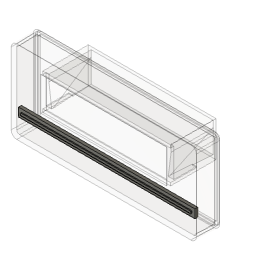
AmigaGotekEnclosure (Autodesk Fusion 360 design; units mm, degrees)
Autodesk Fusion 360 part; units mm, degrees
note: some values were not read from the file. Set by a fixed rule: which face or edge a step refers to.
sketch "Sketch1" plane through (0, 0, 0) normal (0, 1, 0) x (1, 0, 0) in component "face"
  line L0 (77.7875, 34.925) -> (-77.7875, 34.925)
  line L1 (-77.7875, 34.925) -> (-77.7875, -34.925)
  line L2 (-77.7875, -34.925) -> (77.7875, -34.925)
  line L3 (77.7875, -34.925) -> (77.7875, 34.925)
  line L4 (77.7875, 34.925) -> (-77.7875, -34.925) construction
  line L5 (-77.7875, 34.925) -> (77.7875, -34.925) construction
  dimension "d29" = 155.575
  dimension "d30" = 69.85
  constraint horizontal L0
  constraint perpendicular L0 L1
  constraint parallel L0 L2
  constraint parallel L1 L3
  constraint coincident L4 origin
  constraint coincident L5 origin
  measures "d29" distance of L1.end L2.end
  measures "d30" distance of L0.end L1.end
extrude "Extrude1" add sketch "Sketch1" against normal blind 19.05 draft -1 makes body 1 in component "face"
fillet "Fillet1" radius 4.572 4 edges at (-77.6212, -9.525, 34.7587) (77.6212, -9.525, 34.7587) (77.6212, -9.525, -34.7587) (-77.6212, -9.525, -34.7587) on bodies 1 in component "face"
shell "Shell1" thickness 2.3813 removed faces 1 at (-24.4054, 0, -11.6417) on bodies 1 in component "face"
sketch "Sketch2" plane through (0, -19.05, 0) normal (0, -1, 0) x (1, 0, 0) in component "face"
  ellipse E0 centre (-72.8823, -30.0198) end of major axis (-76.1162, -33.2537) minor radius 4.572 (-77.455, -30.0212) -> (-72.8837, -34.5925) ccw
  line L0 (-72.8837, -34.5925) -> (72.8837, -34.5925)
  ellipse E1 centre (72.8823, -30.0198) end of major axis (76.1162, -33.2537) minor radius 4.572 (72.8837, -34.5925) -> (77.455, -30.0212) ccw
  line L1 (77.455, -30.0212) -> (77.455, 30.0212)
  ellipse E2 centre (72.8823, 30.0198) end of major axis (76.1162, 33.2537) minor radius 4.572 (77.455, 30.0212) -> (72.8837, 34.5925) ccw
  line L2 (72.8837, 34.5925) -> (-72.8837, 34.5925)
  ellipse E3 centre (-72.8823, 30.0198) end of major axis (-76.1162, 33.2537) minor radius 4.572 (-72.8837, 34.5925) -> (-77.455, 30.0212) ccw
  line L3 (-77.455, 30.0212) -> (-77.455, -30.0212)
  line L4 (71.4375, -17.5269) -> (-71.4375, -17.5269)
  line L5 (-71.4375, -17.5269) -> (-71.4375, -15.1456)
  line L6 (-71.4375, -15.1456) -> (71.4375, -15.1456)
  line L7 (71.4375, -15.1456) -> (71.4375, -17.5269)
  line L8 (71.4375, -17.5269) -> (-71.4375, -15.1456) construction
  line L9 (-71.4375, -17.5269) -> (71.4375, -15.1456) construction
  line L10 (6.2218, -34.5925) -> (6.2218, -17.5269) construction
  point P0 (0, -16.3362)
  dimension "d36" = 142.875
  dimension "d37" = 2.3813
  dimension "d38" = 17.0656
  constraint horizontal L4
  constraint perpendicular L4 L5
  constraint parallel L4 L6
  constraint parallel L5 L7
  constraint coincident L8 P0
  constraint coincident L9 P0
  constraint coincident L0 L10.start
  constraint coincident L4 L10.end
  constraint perpendicular L4 L10
  measures "d36" distance of L5.end L6.end
  measures "d37" distance of L4.end L5.end
  measures "d38" distance of L10.start L10.end
extrude "Extrude2" cut sketch "Sketch2" against normal up to surface (2.3813 mm away) contours L4 L5 L6 L7 bodies 1 in component "face"
sketch "Sketch3" plane through (0, -16.6688, 0) normal (0, 1, 0) x (-1, 0, 0) in component "face"
  line L0 (-71.4375, -17.5269) -> (-71.4375, -15.1456)
  line L1 (-71.4375, -15.1456) -> (71.4375, -15.1456)
  line L2 (71.4375, -15.1456) -> (71.4375, -17.5269)
  line L3 (71.4375, -17.5269) -> (-71.4375, -17.5269)
  ellipse E0 centre (72.9238, -30.0613) end of major axis (74.4734, -31.6109) minor radius 2.1907 (72.9245, -32.2524) -> (75.1149, -30.062) ccw
  line L4 (75.1149, -30.062) -> (75.1149, 30.062)
  ellipse E1 centre (72.9238, 30.0613) end of major axis (74.4734, 31.6109) minor radius 2.1907 (75.1149, 30.062) -> (72.9245, 32.2524) ccw
  line L5 (72.9245, 32.2524) -> (-72.9245, 32.2524)
  ellipse E2 centre (-72.9238, 30.0613) end of major axis (-74.4734, 31.6109) minor radius 2.1907 (-72.9245, 32.2524) -> (-75.1149, 30.062) ccw
  line L6 (-75.1149, 30.062) -> (-75.1149, -30.062)
  ellipse E3 centre (-72.9238, -30.0613) end of major axis (-74.4734, -31.6109) minor radius 2.1907 (-75.1149, -30.062) -> (-72.9245, -32.2524) ccw
  line L7 (-72.9245, -32.2524) -> (72.9245, -32.2524)
  line L8 (0, -15.1456) -> (0, 32.2524) construction
  line L9 (53.4352, -6.3294) -> (-53.4352, -6.3294)
  line L10 (-53.4352, -6.3294) -> (-53.4352, 23.4362)
  line L11 (-53.4352, 23.4362) -> (53.4353, 23.4362)
  line L12 (53.4353, 23.4362) -> (53.4352, -6.3294)
  line L13 (53.4352, -6.3294) -> (-53.4352, 23.4362) construction
  line L14 (-53.4352, -6.3294) -> (53.4353, 23.4362) construction
  point P0 (0, 8.5534)
  dimension "d42" = 106.8705
  dimension "d43" = 29.7656
  constraint midpoint L1 L8.start
  constraint midpoint L5 L8.end
  constraint horizontal L9
  constraint perpendicular L9 L10
  constraint parallel L9 L11
  constraint parallel L10 L12
  constraint coincident L13 P0
  constraint coincident L14 P0
  constraint midpoint L8 P0
  measures "d42" distance of L10.end L11.end
  measures "d43" distance of L9.end L10.end
extrude "Extrude3" add sketch "Sketch3" along normal blind 38.1 contours L9 L10 L11 L12 bodies 1 in component "face"
shell "Shell2" thickness 2.3813 removed faces 1 at (-17.8118, 21.4312, 13.5144) on bodies 1 in component "face"
ref_plane "WorkPlane4" through (53.4352, 2.3812, 8.5534) normal (1, 0, 0) x (0, 0, -1) in component "face"
sketch "Sketch8" plane through (53.4352, 0, 0) normal (1, 0, 0) x (0, 1, 0) in component "face"
  line L0 (-16.6688, 23.4362) -> (-16.6688, -6.3294)
  line L1 (-16.6688, -6.3294) -> (-16.6688, 23.4362)
  line L2 (-16.6688, -17.5269) -> (-16.6688, -15.1456)
  line L3 (-16.6688, -15.1456) -> (-16.6688, -17.5269)
  line L4 (-16.6688, -32.2524) -> (-16.6688, -30.062)
  line L5 (-16.6688, -30.062) -> (-16.6688, 30.062)
  line L6 (-16.6688, 30.062) -> (-16.6688, 32.2524)
  line L7 (-16.6688, 30.062) -> (-16.6688, 32.2524)
  line L8 (-16.6688, 30.062) -> (-16.6688, -30.062)
  line L9 (-16.6688, -32.2524) -> (-16.6688, -30.062)
  line L10 (-16.6688, -3.9481) -> (21.4312, -3.9481)
  line L11 (21.4312, -3.9481) -> (-16.6688, -3.9481)
  line L12 (-16.6688, 21.055) -> (21.4312, 21.055)
  line L13 (21.4312, 21.055) -> (-16.6688, 21.055)
  line L14 (-16.6688, 21.055) -> (-13.8906, 21.055)
  line L15 (-13.8906, 21.055) -> (-13.8906, -3.9481)
  line L16 (-13.8906, -3.9481) -> (-16.6688, -3.9481)
  line L17 (-16.6688, -3.9481) -> (-16.6688, 21.055)
  dimension "d60" = 2.7781
  constraint horizontal L14
  constraint vertical L15
  constraint horizontal L16
  constraint vertical L17
  constraint coincident L12.start L13.end
  measures "d60" distance of L12.start L14.end
extrude "Extrude6" cut sketch "Sketch8" against normal up to surface (106.8705 mm away) bodies 1 in component "face"
ref_plane "WorkPlane5" through (0, 2.3812, -3.9481) normal (0, 0, 1) x (1, 0, 0) in component "face"
sketch "Sketch9" plane through (0, 0, -3.9481) normal (0, 0, 1) x (1, 0, 0) in component "face"
  line L0 (-51.054, -13.8906) -> (-51.054, 21.4312) construction
  line L1 (-51.054, 21.4312) -> (-51.054, -13.8906) construction
  line L2 (51.054, -13.8906) -> (51.054, 21.4312) construction
  line L3 (51.054, 21.4312) -> (51.054, -13.8906) construction
  line L4 (-51.054, -13.8906) -> (51.054, -13.8906) construction
  line L5 (0, -13.8906) -> (0, 16.5449) construction
  line L6 (-51.054, -13.8906) -> (-48.6728, -13.8906)
  line L7 (-48.6728, -13.8906) -> (-51.054, 21.4312)
  line L8 (-51.054, 21.4312) -> (-51.054, -13.8906)
  line L9 (51.054, -13.8906) -> (48.6727, -13.8906)
  line L10 (48.6727, -13.8906) -> (51.054, 21.4313)
  line L11 (51.054, 21.4313) -> (51.054, -13.8906)
  dimension "d64" = 2.3813
  constraint coincident L0.start L1.end
  constraint coincident L2.start L3.end
  constraint midpoint L4 L5.start
  constraint perpendicular L4 L5
  constraint perpendicular L0 L6
  constraint coincident L0.end L1.start
  constraint symmetric L5 L0.start L2.start
  constraint symmetric L5 L6.end L9.end
  constraint symmetric L5 L0.end L10.end
  measures "d64" distance of L0.start L6.end
extrude "Extrude7" add sketch "Sketch9" along normal up to surface (25.0031 mm away) bodies 1 in component "face"
ref_plane "WorkPlane6" through (-51.054, -13.8906, 8.5534) normal (0, -1, 0) x (0, 0, 1) in component "face"
sketch "Sketch10" plane through (0, -13.8906, 0) normal (0, -1, 0) x (-1, 0, 0) in component "face"
  line L0 (51.054, -21.055) -> (48.6728, -21.055)
  line L1 (48.6728, -21.055) -> (48.6728, 3.9481)
  line L2 (48.6728, 3.9481) -> (51.054, 3.9481)
  line L3 (51.054, 3.9481) -> (51.054, -21.055)
  line L4 (-48.6727, -21.055) -> (-51.054, -21.055)
  line L5 (-51.054, -21.055) -> (-51.054, 3.9481)
  line L6 (-51.054, 3.9481) -> (-48.6727, 3.9481)
  line L7 (-48.6727, 3.9481) -> (-48.6727, -21.055)
  line L8 (51.054, 3.9481) -> (48.6728, 3.9481)
  line L9 (48.6728, 3.9481) -> (53.4352, 3.9481)
  line L10 (53.4352, 3.9481) -> (-53.4352, 3.9481)
  line L11 (-53.4352, 3.9481) -> (-48.6727, 3.9481)
  line L12 (-48.6727, 3.9481) -> (-51.054, 3.9481)
  line L13 (-51.054, 3.9481) -> (51.054, 3.9481)
  line L14 (48.6728, -21.055) -> (51.054, -21.055)
  line L15 (51.054, -21.055) -> (-51.054, -21.055)
  line L16 (-51.054, -21.055) -> (-48.6727, -21.055)
  line L17 (-48.6727, -21.055) -> (-53.4352, -21.055)
  line L18 (-53.4352, -21.055) -> (53.4353, -21.055)
  line L19 (53.4353, -21.055) -> (48.6728, -21.055)
  line L20 (53.4352, 3.9481) -> (53.4353, -21.055)
  line L21 (53.4353, -21.055) -> (53.4353, -23.4362)
  line L22 (53.4353, -23.4362) -> (53.4352, 6.3294)
  line L23 (53.4352, 6.3294) -> (53.4352, 3.9481)
  line L24 (-53.4352, -21.055) -> (-53.4352, 3.9481)
  line L25 (-53.4352, 3.9481) -> (-53.4352, 6.3294)
  line L26 (-53.4352, 6.3294) -> (-53.4352, -23.4362)
  line L27 (-53.4352, -23.4362) -> (-53.4352, -21.055)
  line L28 (48.6728, 3.9481) -> (-48.6727, 3.9481) construction
  line L29 (0, 3.9481) -> (0, -21.055) construction
  line L30 (51.054, 3.9481) -> (51.054, -15.4987) construction
  line L31 (51.054, -15.4987) -> (48.6728, 3.9481)
  line L32 (48.6728, 3.9481) -> (48.6728, -21.055)
  line L33 (48.6728, -21.055) -> (51.054, -21.055)
  line L34 (51.054, -21.055) -> (51.054, -15.4987)
  line L35 (-48.6728, -21.055) -> (-51.054, -21.055)
  line L36 (-48.6727, 3.9481) -> (-48.6728, -21.055)
  line L37 (-51.054, -21.055) -> (-51.054, -15.4987)
  line L38 (-51.054, -15.4987) -> (-48.6727, 3.9481)
  dimension "d68" = 19.4469
  constraint coincident L1.end L2.start
  constraint coincident L6.end L7.start
  constraint midpoint L28 L29.start
  constraint midpoint L18 L29.end
  constraint coincident L2.end L3.start
  constraint perpendicular L8 L30
  constraint coincident L0.end L1.start
  constraint coincident L0.start L3.end
  constraint symmetric L1.end L29 L6.end
  constraint symmetric L29 L30.end L37.end
  constraint symmetric L29 L1.end L6.end
  constraint symmetric L29 L0.end L35.start
  constraint symmetric L29 L0.start L4.end
  measures "d68" distance of L2.end L30.end
extrude "Extrude8" cut sketch "Sketch10" against normal up to surface (35.3219 mm away) contours L0 L1 L3 L14 L15 L18 L19 L31 L32 L33 L34 | L4 L5 L7 L15 L16 L17 L18 L35 L36 L37 L38 bodies 1 in component "face"
sketch "Sketch11" plane through (53.4352, 0, 0) normal (1, 0, 0) x (0, 1, 0) in component "face"
  line L0 (-16.6688, 21.055) -> (-13.8906, 21.055)
  line L1 (-13.8906, 21.055) -> (-13.8906, -3.9481)
  line L2 (-13.8906, -3.9481) -> (-16.6688, -3.9481)
  line L3 (-16.6688, -3.9481) -> (-16.6688, -6.3294)
  line L4 (-16.6688, -6.3294) -> (21.4312, -6.3294)
  line L5 (21.4312, -6.3294) -> (21.4312, 23.4362)
  line L6 (21.4312, 23.4362) -> (-16.6688, 23.4362)
  line L7 (-16.6688, 23.4362) -> (-16.6688, 21.055)
  line L8 (-13.8906, -3.9481) -> (21.4312, -3.9481)
  line L9 (21.4313, -3.9481) -> (-13.8906, -3.9481)
  line L10 (-13.8906, -3.9481) -> (-16.6687, -3.9481)
  line L11 (-16.6688, -3.9481) -> (-13.8906, -3.9481)
  line L12 (-13.8906, 21.055) -> (-13.8906, 15.4987)
  line L13 (-13.8906, 15.4987) -> (-13.8906, -3.9481)
  line L14 (-13.8906, -3.9481) -> (-13.8906, 21.055)
  line L15 (-13.8906, -3.9481) -> (5.1594, -3.9481)
  line L16 (5.1594, -3.9481) -> (5.1594, -3.1544)
  line L17 (5.1594, -3.1544) -> (-13.8906, -3.1544)
  line L18 (-13.8906, -3.1544) -> (-13.8906, -3.9481)
  dimension "d73" = 19.05
  dimension "d74" = 0.7937
  constraint horizontal L15
  constraint vertical L16
  constraint horizontal L17
  constraint vertical L18
  constraint coincident L1.end L2.start
  measures "d73" distance of L1.end L15.end
  measures "d74" distance of L1.end L17.end
extrude "Extrude9" cut sketch "Sketch11" against normal up to surface (106.8705 mm away) contours L1 L8 L9 L13 L14 L15 L16 L17 L18 bodies 1 in component "face"
ref_plane "WorkPlane7" through (0, -16.6688, 0) normal (0, 1, 0) x (1, 0, 0) in component "face"
sketch "Sketch14" plane through (0, -16.6688, 0) normal (0, 1, 0) x (1, 0, 0) in component "face"
  line L0 (51.054, -21.055) -> (51.054, -15.4987)
  line L1 (51.054, -15.4987) -> (51.054, -21.055)
  line L2 (51.054, -21.055) -> (53.4352, -21.055)
  line L3 (53.4352, -21.055) -> (-53.4353, -21.055)
  line L4 (-53.4353, -21.055) -> (-51.054, -21.055)
  line L5 (-51.054, -21.055) -> (51.054, -21.055)
  line L6 (-51.054, -15.4987) -> (-51.054, -21.055)
  line L7 (-51.054, -21.055) -> (-51.054, -15.4987)
  line L8 (49.957, 3.9481) -> (51.054, 3.9481)
  line L9 (51.054, 3.9481) -> (-51.054, 3.9481)
  line L10 (-51.054, 3.9481) -> (-49.957, 3.9481)
  line L11 (-49.957, 3.9481) -> (-53.4352, 3.9481)
  line L12 (-53.4352, 3.9481) -> (53.4352, 3.9481)
  line L13 (53.4352, 3.9481) -> (49.957, 3.9481)
  line L14 (51.054, -21.055) -> (-51.054, -21.055) construction
  line L15 (-51.054, -21.055) -> (-51.054, 3.9481) construction
  line L16 (-51.054, 3.9481) -> (51.054, 3.9481) construction
  line L17 (51.054, 3.9481) -> (51.054, -21.055) construction
  line L18 (-50.2602, -20.2612) -> (-50.2602, 3.1544)
  line L19 (-50.2602, 3.1544) -> (50.2603, 3.1544)
  line L20 (50.2603, 3.1544) -> (50.2603, -20.2612)
  line L21 (50.2603, -20.2612) -> (-50.2602, -20.2612)
  dimension "d81" = 0.7937
  constraint horizontal L14
  constraint vertical L15
  constraint horizontal L16
  constraint vertical L17
  constraint coincident L9.end L10.start
  constraint coincident L0.start L1.end
extrude "Extrude10" cut sketch "Sketch14" against normal up to surface (2.3812 mm away) bodies 1 in component "face"
ref_plane "WorkPlane8" through (0, 0, 0) normal (1, 0, 0) x (0, 1, 0) in component "face"
sketch "Sketch15" plane through (0, 0, 0) normal (1, 0, 0) x (0, 1, 0) in component "face"
  line L0 (-19.05, -3.1544) -> (-16.6688, -3.1544)
  line L1 (-16.6688, -3.1544) -> (-19.05, -3.1544)
  line L2 (-16.6688, 20.2612) -> (-16.6688, -3.1544)
  line L3 (-16.6688, -3.1544) -> (-16.6688, 20.2612)
  line L4 (-16.6688, -3.9481) -> (-16.6688, -6.3294)
  line L5 (-16.6688, -6.3294) -> (-16.6688, -3.9481)
  line L6 (-16.6688, -32.2524) -> (-16.6688, -30.062)
  line L7 (-16.6688, -30.062) -> (-16.6688, 30.062)
  line L8 (-16.6688, 30.062) -> (-16.6688, 32.2524)
  line L9 (-16.6688, 30.062) -> (-16.6688, 32.2524)
  line L10 (-16.6688, 30.062) -> (-16.6688, -30.062)
  line L11 (-16.6688, -32.2524) -> (-16.6688, -30.062)
  line L12 (-16.6688, -17.5269) -> (-16.6688, -15.1456)
  line L13 (-16.6688, -15.1456) -> (-16.6688, -17.5269)
  line L14 (-16.6688, 21.055) -> (-16.6688, 23.4362)
  line L15 (-16.6688, 23.4362) -> (-16.6688, 21.055)
  line L16 (-16.6688, -3.1544) -> (-19.05, -3.1544)
  line L17 (-19.05, -3.1544) -> (-19.05, -5.5356)
  line L18 (-19.05, -5.5356) -> (-16.6688, -3.1544)
  constraint coincident L0.end L1.start
  constraint coincident L0.start L1.end
  constraint perpendicular L1 L17
  constraint equal L16 L17
sweep "Sweep1" cut profiles "Sketch15" along 4 edges at (0, -16.6688, 20.2612) (-50.2602, -16.6688, 8.5534) (0, -16.6688, -3.1544) (50.2603, -16.6688, 8.5534) section 1 on bodies 1 bodies 1 in component "face"
sketch "Sketch16" plane through (0, 0, 0) normal (0, 1, 0) x (-1, 0, 0) in component "face"
  ellipse E0 centre (73.2148, -30.3523) end of major axis (74.7644, -31.9019) minor radius 2.1907 (73.2155, -32.5434) -> (75.4059, -30.353) ccw
  line L0 (73.2155, -32.5434) -> (-73.2155, -32.5434)
  ellipse E1 centre (-73.2148, -30.3523) end of major axis (-74.7644, -31.9019) minor radius 2.1907 (-75.4059, -30.353) -> (-73.2155, -32.5434) ccw
  line L1 (-75.4059, -30.353) -> (-75.4059, 30.353)
  ellipse E2 centre (-73.2148, 30.3523) end of major axis (-74.7644, 31.9019) minor radius 2.1907 (-73.2155, 32.5434) -> (-75.4059, 30.353) ccw
  line L2 (-73.2155, 32.5434) -> (73.2155, 32.5434)
  ellipse E3 centre (73.2148, 30.3523) end of major axis (74.7644, 31.9019) minor radius 2.1907 (75.4059, 30.353) -> (73.2155, 32.5434) ccw
  line L3 (75.4059, 30.353) -> (75.4059, -30.353)
  ellipse E4 centre (73.2148, -30.3523) end of major axis (76.4487, -33.5862) minor radius 4.572 (73.2162, -34.925) -> (77.7875, -30.3537) ccw
  line L4 (77.7875, -30.3537) -> (77.7875, 30.3537)
  ellipse E5 centre (73.2148, 30.3523) end of major axis (76.4487, 33.5862) minor radius 4.572 (77.7875, 30.3537) -> (73.2162, 34.925) ccw
  line L5 (73.2162, 34.925) -> (-73.2162, 34.925)
  ellipse E6 centre (-73.2148, 30.3523) end of major axis (-76.4487, 33.5862) minor radius 4.572 (-73.2162, 34.925) -> (-77.7875, 30.3537) ccw
  line L6 (-77.7875, 30.3537) -> (-77.7875, -30.3537)
  ellipse E7 centre (-73.2148, -30.3523) end of major axis (-76.4487, -33.5862) minor radius 4.572 (-77.7875, -30.3537) -> (-73.2162, -34.925) ccw
  line L7 (-73.2162, -34.925) -> (73.2162, -34.925)
  line L8 (-77.7875, 30.3537) -> (-77.7875, -30.3537)
  ellipse E8 centre (-73.2148, 30.3523) end of major axis (-76.4487, 33.5862) minor radius 4.572 (-73.2162, 34.925) -> (-77.7875, 30.3537) ccw
  line L9 (73.2162, 34.925) -> (-73.2162, 34.925)
  ellipse E9 centre (-73.2148, -30.3523) end of major axis (-76.4487, -33.5862) minor radius 4.572 (-77.7875, -30.3537) -> (-73.2162, -34.925) ccw
  line L10 (-73.2162, -34.925) -> (73.2162, -34.925)
  ellipse E10 centre (73.2148, -30.3523) end of major axis (76.4487, -33.5862) minor radius 4.572 (73.2162, -34.925) -> (77.7875, -30.3537) ccw
  line L11 (77.7875, -30.3537) -> (77.7875, 30.3537)
  ellipse E11 centre (73.2148, 30.3523) end of major axis (76.4487, 33.5862) minor radius 4.572 (77.7875, 30.3537) -> (73.2162, 34.925) ccw
  line L12 (-73.2162, -33.3375) -> (73.2162, -33.3375)
  spline S0 degree 3 poles (73.2162, -33.3375) (74.2378, -33.3375) (75.241, -32.7718) (75.7695, -31.8978) (76.0494, -31.435) (76.2, -30.8948) (76.2, -30.3537) knots -0.785246 -0.785246 -0.785246 -0.785246 0.241471 0.241471 0.241471 0.785246 0.785246 0.785246 0.785246
  line L13 (76.2, -30.3537) -> (76.2, 30.3537)
  spline S1 degree 3 poles (76.2, 30.3537) (76.2, 31.3753) (75.6343, 32.3785) (74.7603, 32.907) (74.2975, 33.1869) (73.7573, 33.3375) (73.2162, 33.3375) knots -0.785246 -0.785246 -0.785246 -0.785246 0.241471 0.241471 0.241471 0.785246 0.785246 0.785246 0.785246
  line L14 (73.2162, 33.3375) -> (-73.2162, 33.3375)
  spline S2 degree 3 poles (-73.2162, 33.3375) (-74.2378, 33.3375) (-75.241, 32.7718) (-75.7695, 31.8978) (-76.0494, 31.435) (-76.2, 30.8948) (-76.2, 30.3537) knots -0.785246 -0.785246 -0.785246 -0.785246 0.241471 0.241471 0.241471 0.785246 0.785246 0.785246 0.785246
  line L15 (-76.2, 30.3537) -> (-76.2, -30.3537)
  spline S3 degree 3 poles (-76.2, -30.3537) (-76.2, -31.3753) (-75.6343, -32.3785) (-74.7603, -32.907) (-74.2975, -33.1869) (-73.7573, -33.3375) (-73.2162, -33.3375) knots -0.785246 -0.785246 -0.785246 -0.785246 0.241471 0.241471 0.241471 0.785246 0.785246 0.785246 0.785246
  line L16 (-73.2162, -30.9562) -> (73.2162, -30.9562)
  spline S4 degree 3 poles (73.2162, -30.9562) (73.5324, -30.9562) (73.8188, -30.6699) (73.8188, -30.3537) knots -0.785246 -0.785246 -0.785246 -0.785246 0.785246 0.785246 0.785246 0.785246
  line L17 (73.8188, -30.3537) -> (73.8188, 30.3537)
  spline S5 degree 3 poles (73.8188, 30.3537) (73.8188, 30.6699) (73.5324, 30.9562) (73.2162, 30.9562) knots -0.785246 -0.785246 -0.785246 -0.785246 0.785246 0.785246 0.785246 0.785246
  line L18 (73.2162, 30.9562) -> (-73.2162, 30.9562)
  spline S6 degree 3 poles (-73.2162, 30.9562) (-73.5324, 30.9562) (-73.8188, 30.6699) (-73.8188, 30.3537) knots -0.785246 -0.785246 -0.785246 -0.785246 0.785246 0.785246 0.785246 0.785246
  line L19 (-73.8188, 30.3537) -> (-73.8188, -30.3537)
  spline S7 degree 3 poles (-73.8188, -30.3537) (-73.8188, -30.6699) (-73.5324, -30.9562) (-73.2162, -30.9562) knots -0.785246 -0.785246 -0.785246 -0.785246 0.785246 0.785246 0.785246 0.785246
extrude "Extrude12" add sketch "Sketch16" along normal blind 1.5875 contours E0 L0 E1 L1 E2 L2 E3 L3 | L12 S0 L13 S1 L14 S2 L15 S3 bodies 1 in component "face"
sketch "Sketch17" plane through (53.4352, 0, 0) normal (1, 0, 0) x (0, 1, 0) in component "face"
  line L0 (0, -30.9563) -> (0, -30.3537)
  line L1 (0, -30.3537) -> (0, -30.9563)
  line L2 (0, -30.3537) -> (0, 30.3537)
  line L3 (0, 30.9563) -> (0, 30.3537)
  line L4 (0, 30.3537) -> (0, 30.9563)
  line L5 (0, 30.3537) -> (0, -30.3537)
  line L6 (0, -30.353) -> (0, -32.5434)
  line L7 (0, -30.353) -> (0, -32.5434)
  line L8 (0, -30.353) -> (0, 30.353)
  line L9 (0, 32.5434) -> (0, 30.353)
  line L10 (0, 32.5434) -> (0, 30.353)
  line L11 (0, 30.353) -> (0, -30.353)
  line L12 (0, -32.5434) -> (-16.6688, -32.2524)
  line L13 (-16.6688, -32.2524) -> (0, -32.5434)
  line L14 (0, -30.9563) -> (0, -32.5434)
  line L15 (0, -32.5434) -> (-1.5869, -32.5157)
  line L16 (0, -30.9563) -> (-1.5869, -32.5157)
  constraint coincident L0.start L1.end
  constraint coincident L6.end L7.end
  constraint coincident L13 L15.end
  constraint parallel L13 L15
  constraint equal L14 L15
sweep "Sweep2" add profiles "Sketch17" along 8 edges at (75.4059, 0, 0) (74.7644, 0, 31.9019) (0, 0, 32.5434) (-74.7644, 0, 31.9019) (-75.4059, 0, 0) (-74.7644, 0, -31.9019) (0, 0, -32.5434) (74.7644, 0, -31.9019) section 1 on bodies 1 bodies 1 in component "face"
sketch "Sketch1 (2)" plane through (0, -16.6688, 0) normal (0, 1, 0) x (-1, 0, 0) in component "accent_line"
  line L0 (-50.2603, 20.2612) -> (50.2602, 20.2612)
  line L1 (50.2602, 20.2612) -> (50.2602, -3.1544)
  line L2 (50.2602, -3.1544) -> (-50.2603, -3.1544)
  line L3 (-50.2603, -3.1544) -> (-50.2603, 20.2612)
  line L4 (-53.4352, -3.9481) -> (53.4352, -3.9481)
  line L5 (53.4352, -3.9481) -> (53.4352, -6.3294)
  line L6 (53.4352, -6.3294) -> (-53.4352, -6.3294)
  line L7 (-53.4352, -6.3294) -> (-53.4352, -3.9481)
  ellipse E0 centre (72.9238, -30.0613) end of major axis (74.4734, -31.6109) minor radius 2.1907 (72.9245, -32.2524) -> (75.1149, -30.062) ccw
  line L8 (75.1149, -30.062) -> (75.1149, 30.062)
  ellipse E1 centre (72.9238, 30.0613) end of major axis (74.4734, 31.6109) minor radius 2.1907 (75.1149, 30.062) -> (72.9245, 32.2524) ccw
  line L9 (72.9245, 32.2524) -> (-72.9245, 32.2524)
  ellipse E2 centre (-72.9238, 30.0613) end of major axis (-74.4734, 31.6109) minor radius 2.1907 (-72.9245, 32.2524) -> (-75.1149, 30.062) ccw
  line L10 (-75.1149, 30.062) -> (-75.1149, -30.062)
  ellipse E3 centre (-72.9238, -30.0613) end of major axis (-74.4734, -31.6109) minor radius 2.1907 (-75.1149, -30.062) -> (-72.9245, -32.2524) ccw
  line L11 (-72.9245, -32.2524) -> (72.9245, -32.2524)
  line L12 (-71.4375, -17.5269) -> (-71.4375, -15.1456)
  line L13 (-71.4375, -15.1456) -> (71.4375, -15.1456)
  line L14 (71.4375, -15.1456) -> (71.4375, -17.5269)
  line L15 (71.4375, -17.5269) -> (-71.4375, -17.5269)
  line L16 (53.4353, 21.055) -> (-53.4352, 21.055)
  line L17 (-53.4352, 21.055) -> (-53.4352, 23.4362)
  line L18 (-53.4352, 23.4362) -> (53.4353, 23.4362)
  line L19 (53.4353, 23.4362) -> (53.4353, 21.055)
  line L20 (-71.4375, -15.1456) -> (71.4375, -15.1456)
  line L21 (-71.4375, -17.5269) -> (-71.4375, -15.1456)
  line L22 (71.4375, -15.1456) -> (71.4375, -17.5269)
  line L23 (71.4375, -17.5269) -> (-71.4375, -17.5269)
  line L24 (-71.4375, -15.1456) -> (71.4375, -15.1456)
  line L25 (71.4375, -15.1456) -> (71.4375, -17.5269)
  line L26 (71.4375, -17.5269) -> (-71.4375, -17.5269)
  line L27 (-71.4375, -17.5269) -> (-71.4375, -15.1456)
  line L28 (71.1835, -17.2729) -> (-71.1835, -17.2729)
  line L29 (-71.1835, -17.2729) -> (-71.1835, -15.3996)
  line L30 (-71.1835, -15.3996) -> (71.1835, -15.3996)
  line L31 (71.1835, -15.3996) -> (71.1835, -17.2729)
  line L32 (73.8187, -19.9081) -> (-73.8188, -19.9081)
  line L33 (-73.8188, -19.9081) -> (-73.8188, -12.7644)
  line L34 (-73.8188, -12.7644) -> (73.8187, -12.7644)
  line L35 (73.8187, -12.7644) -> (73.8187, -19.9081)
  dimension "d108" = 0.254
  constraint horizontal L24
  constraint vertical L25
  constraint horizontal L26
  constraint vertical L27
  constraint coincident L14.end L15.start
  constraint coincident L12.end L13.start
extrude "Extrude1'" add sketch "Sketch1 (2)" against normal blind 0.7937 separate body contours L28 L29 L30 L31 makes body 2 in component "accent_line"
extrude "Extrude2'" add sketch "Sketch1 (2)" along normal blind 2.3813 contours L12 L13 L14 L15 L20 L21 L22 L23 L24 L25 L26 L27 | L28 L29 L30 L31 | L32 L33 L34 L35 bodies 2 in component "accent_line"
component "face" placed x (1, 0, 0) y (0, 1, 0) z (0, 0, 1) at (0, 0, 0)
component "accent_line" placed x (1, 0, 0) y (0, 1, 0) z (0, 0, 1) at (0, 0, 0)
equation "accent_line_bottom_offset = 43/64\"" comment "Face accent line distance from bottom"
equation "accent_line_height = 3/32\"" comment "Face accent line height"
equation "accent_line_width = enclosure_width - 1/2\"" comment "Face accent line height"
equation "enclosure_corner_radius = 0.18 in" comment "Corner radius for enclosure"
equation "enclosure_depth = 8 1/2\"" comment "Overall enclosure depth"
equation "enclosure_height = 2 3/4\"" comment "Overall enclosure height"
equation "enclosure_width = 6 1/8\"" comment "Overall enclosure width"
equation "face_depth = 3/4\"" comment "Face component depth"
equation "face_extrude_angle = 1 deg" comment "Face component extrude angle"
equation "gotek_mount_sleeve_depth = 1 1/2\"" comment "Gotek drive mounting sleeve depth"
equation "gotek_mount_sleeve_face_depth = 7/64\"" comment "Gotek drive face depth used to lock into mounting sleeve"
equation "gotek_mount_sleeve_height = 63/64\"" comment "Gotek drive mounting sleeve height"
equation "gotek_mount_sleeve_latch_height = 49/64\"" comment "Gotek drive mounting sleeve latch height"
equation "gotek_mount_sleeve_latch_width = 3/32\"" comment "Gotek drive mounting sleeve latch width"
equation "gotek_mount_sleeve_width = 4.02 in" comment "Gotek drive mounting sleeve width"
equation "shell_thickness = 3/32\"" comment "Overall enclosure shell thickness"
equation "d29 = enclosure_width"
equation "d30 = enclosure_height"
equation "d31 = -face_depth"
equation "d32 = -face_extrude_angle"
equation "d34 = enclosure_corner_radius"
equation "d35 = shell_thickness"
equation "d36 = accent_line_width"
equation "d37 = accent_line_height"
equation "d38 = accent_line_bottom_offset"
equation "d39 = 0\""
equation "accent_line_depth = 1/16\""
equation "d42 = gotek_mount_sleeve_width + ( shell_thickness * 2 )"
equation "d43 = gotek_mount_sleeve_height + ( shell_thickness * 2 )"
equation "d44 = gotek_mount_sleeve_depth"
equation "d46 = shell_thickness"
equation "d59 = 0\""
equation "d60 = gotek_mount_sleeve_face_depth"
equation "d61 = 0\""
equation "d63 = 0\""
equation "d64 = gotek_mount_sleeve_latch_width"
equation "d65 = 0\""
equation "d67 = 0\""
equation "d68 = gotek_mount_sleeve_latch_height"
equation "d69 = 0\""
equation "gotek_mounting_sleeve_latch_bottom_gap_height = 1/32\""
equation "gotek_mounting_sleeve_latch_bottom_gap_depth = gotek_mount_sleeve_depth * 0.5"
equation "d73 = gotek_mounting_sleeve_latch_bottom_gap_depth"
equation "d74 = gotek_mounting_sleeve_latch_bottom_gap_height"
equation "d75 = 0\""
equation "gotek_window_inset = 1/32\""
equation "d80 = 0\""
equation "d81 = gotek_window_inset"
equation "d82 = 0\""
equation "d84 = 0\""
equation "face_seam_inset = 1/16\"" comment "The inset of the seam between the face and the enclsoure body"
equation "face_seam_depth = 1/16\"" comment "The depth of the seam between the face and the enclosure body"
equation "d97 = -face_seam_inset"
equation "d98 = -( shell_thickness + face_seam_inset )"
equation "d99 = face_seam_depth"
equation "accent_line_filler_inset = 0.01 in"
equation "d108 = accent_line_filler_inset"
equation "accent_line_back_offset = shell_thickness"
equation "d110 = -accent_line_back_offset"
equation "accent_line_filler_depth = shell_thickness - 1/16\""
equation "d112 = -accent_line_filler_depth"
equation "d114 = accent_line_back_offset"
named bodies: "face"
